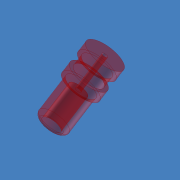
# Autodesk Inventor part: Blende
Saved by Autodesk Inventor 2013 (Build 170138000, 138)
## iProperties
Created: 2007-03-19
Part Number: Blende
Document SubType Name: Modeling
Designer: Administrator
Manufacturer: Standard
Standards Organization: Custom
Material: Allgemein
Density: 1 g/cm^3
Author: Administrator
Autodesk Inventor part; units mm, degrees
ref_plane "YZ Plane" through (0, 0, 0) normal (1, 0, 0) x (0, 1, 0)
ref_plane "XZ Plane" through (0, 0, 0) normal (0, 1, 0) x (-1, 0, 0)
ref_plane "XY Plane" through (0, 0, 0) normal (0, 0, 1) x (1, 0, 0)
sketch "Skizze1" plane through (0, 0, 0) normal (0, 0, 1) x (1, 0, 0)
  line L0 (0, 0.3238) -> (2, 0.3238)
  line L1 (2, 0.3238) -> (2, 0.7238)
  line L2 (2, 0.7238) -> (0.9, 0.7238)
  line L3 (0.9, 0.7238) -> (0.9, 0.8238)
  line L4 (0.9, 0.8238) -> (0.6, 0.8238)
  line L5 (0.6, 0.8238) -> (0.6, 0.7238)
  line L6 (0.6, 0.7238) -> (0.3, 0.7238)
  line L7 (0.3, 0.7238) -> (0.3, 0.8238)
  line L8 (0.3, 0.8238) -> (0, 0.8238)
  line L9 (0, 0.8238) -> (0, 0.3238)
  dimension "d1" = 2
  dimension "d6" = 0.3
  dimension "d7" = 0.3
  dimension "d8" = 0.3
  dimension "d10" = 0.5
  dimension "d11" = 0.4
  constraints: 20 end point, 7 parallel, 2 collinear, 2 perpendicular, 1 horizontal
  measures "d1" distance of L0.start L0.end
  measures "d6" distance of L7.end L8.end
  measures "d7" distance of L5.end L6.end
  measures "d8" distance of L3.end L4.end
  measures "d10" distance of L8.end L0.start
  measures "d11" distance of L0.end L1.end
revolve "Drehung1" add sketch "Skizze1" angle 360 about axis through (0, 0.3238, 0) along (1, 0, 0)
hole "Bohrung1" at (0, 0.3238, 0) direction (1, 0, 0) diameter 0.15 depth 8
hole "Bohrung2" at (2, 0.3238, 0) direction (-1, 0, 0) diameter 0.5 depth 1
fillet "Rundung1" radius 0.1 1 edges at (2, -0.0762, 0)
